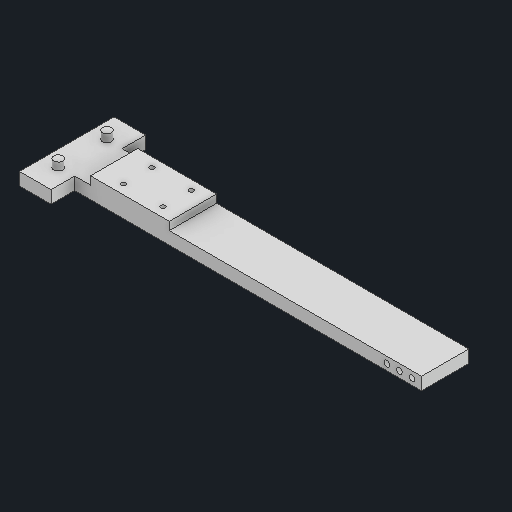
# Autodesk Inventor part: Arm
Saved by Autodesk Inventor 2026.1 (Build 301233020, 233B)
## iProperties
Created: 2025-10-26
Part Number: Arm
Material: Generic
Document SubType Name: Modeling
Designer: Garfieldcmix
Density: 1 g/cm^3
Appearance: Default
Author: Garfieldcmix
Autodesk Inventor part; units mm, degrees
ref_plane "YZ Plane" through (0, 0, 0) normal (1, 0, 0) x (0, 1, 0)
ref_plane "XZ Plane" through (0, 0, 0) normal (0, 1, 0) x (-1, 0, 0)
ref_plane "XY Plane" through (0, 0, 0) normal (0, 0, 1) x (1, 0, 0)
sketch "Sketch1" plane through (0, 0, 0) normal (0, 1, 0) x (-1, 0, 0)
  line L0 (10, 30) -> (10, -30)
  line L1 (10, -30) -> (-10, -30)
  line L2 (-10, -30) -> (-10, -15)
  line L3 (-10, -15) -> (-230, -15)
  line L4 (-230, -15) -> (-230, 15)
  line L5 (-230, 15) -> (-10, 15)
  line L6 (-10, 15) -> (-10, 30)
  line L7 (-10, 30) -> (10, 30)
  line L8 (58, 0) -> (-278, 0) construction
  point P0 (0, 0)
  dimension "d0" = 60
  dimension "d2" = 10
  dimension "d3" = 10
  dimension "d4" = 30
  dimension "d5" = 220
  constraints: 16 end point, 4 symmetric about line, 3 perpendicular, 1 vertical
  measures "d0" distance of L0.start L0.end
  measures "d2" horizontal distance of point (0, 0) L0.end
  measures "d3" horizontal distance of L1.end point (0, 0)
  measures "d4" distance of L3.end L4.end
  measures "d5" distance of L2.end L3.end
extrude "Extrusion1" add sketch "Sketch1" along normal blind 8
sketch "Sketch2" plane through (0, 8, 0) normal (0, 1, 0) x (1, 0, 0)
  circle A0 centre (0, -15.5) radius 2.9
  circle A1 centre (0, 15.5) radius 2.9
  line L0 (0, 42) -> (0, -42) construction
  line L1 (-58, 0) -> (278, 0) construction
  point P0 (0, 0)
  dimension "d8" = 5.8
  dimension "d9" = 31
  constraints: 2 centre point, 2 point on line, 1 equal radius, 1 symmetric about line
  measures "d8" diameter of A0
  measures "d9" distance of A1.centre A0.centre
extrude "Extrusion2" add sketch "Sketch2" along normal blind 4.9
sketch "Sketch3" plane through (0, 8, 0) normal (0, 1, 0) x (1, 0, 0)
  line L0 (230, 15) -> (10, 15) construction
  line L1 (10, -15) -> (230, -15) construction
  line L2 (20, 15) -> (70, 15)
  line L3 (70, 15) -> (70, -15)
  line L4 (70, -15) -> (20, -15)
  line L5 (20, -15) -> (20, 15)
  point P0 (0, 0)
  dimension "d12" = 10
  dimension "d13" = 50
  constraints: 8 end point, 2 parallel, 2 point on line, 1 horizontal, 1 perpendicular
  measures "d12" distance from line of L5 L0.end
  measures "d13" distance of L2.end L2.start
extrude "Extrusion3" add sketch "Sketch3" along normal blind 5.1
sketch "Sketch4" plane through (0, 13.1, 0) normal (0, 1, 0) x (1, 0, 0)
  circle A0 centre (35, 9) radius 1.475
  circle A1 centre (60, 9) radius 1.475
  circle A2 centre (35, -9) radius 1.475
  circle A3 centre (60, -9) radius 1.475
  line L0 (-58, 0) -> (278, 0) construction
  line L1 (35, 9) -> (35, -9) construction
  line L2 (60, 9) -> (60, -9) construction
  line L3 (20, 15) -> (20, -15) construction
  point P0 (0, 0)
  dimension "d16" = 2.95
  dimension "d17" = 18
  dimension "d18" = 25
  dimension "d19" = 15
  constraints: 4 centre point, 4 end point, 3 equal radius, 2 symmetric about line, 2 vertical, 1 parallel
  measures "d16" diameter of A0
  measures "d17" distance of L1.start L1.end
  measures "d18" distance of L2.start L1.start
  measures "d19" distance from line of L3 L1.start
extrude "Extrusion4" cut sketch "Sketch4" against normal up to surface (13.1 mm away)
sketch "Sketch5" plane through (10, 0, 15) normal (0, 0, 1) x (1, 0, 0)
  line L0 (220, 0) -> (220, 8) construction
  line L1 (220, 4) -> (198, 4) construction
  circle A0 centre (198, 4) radius 1.85
  circle A1 centre (214, 4) radius 1.85
  circle A2 centre (206, 4) radius 1.85
  point P0 (-10, 0)
  dimension "d22" = 3.7
  dimension "d23" = 6
  dimension "d25" = 8
  dimension "d26" = 8
  constraints: 3 centre point, 2 end point, 2 equal radius, 2 point on line, 1 coincident, 1 horizontal, 1 midpoint
  measures "d22" diameter of A0
  measures "d23" distance from line of L0 A1.centre
  measures "d25" distance of A2.centre A1.centre
  measures "d26" distance of L1.end A2.centre
extrude "Extrusion5" cut sketch "Sketch5" against normal up to surface (30 mm away)
body "Solid1"
